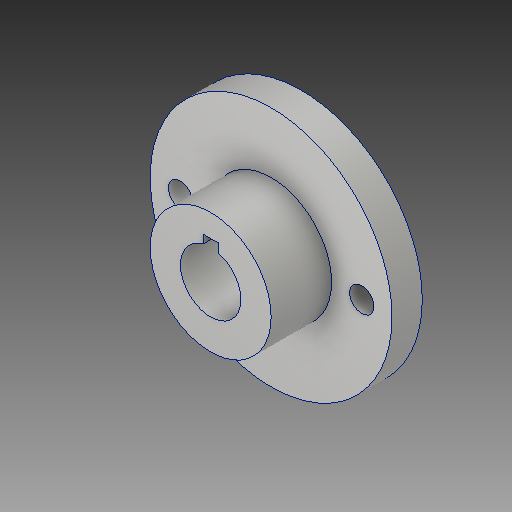
# Autodesk Inventor part: Hub Connected to Steel Tubing - 0.5in. Diameter
Saved by Autodesk Inventor 2019 (Build 230136000, 136)
## iProperties
Created: 2018-11-13
Part Number: Hub Connected to Steel Tubing - 0.5in. Diameter
Material: Aluminum 6061
Document SubType Name: Modeling
Designer: Alex Barnett
Density: 2.7 g/cm^3
Appearance: Aluminum - Flat
Mass: 44.6442 g
Surface Area: 67.6582 cm^2
Volume: 16.5349 cm^3
Author: Alex Barnett
Autodesk Inventor part; units mm, degrees
ref_plane "YZ Plane" through (0, 0, 0) normal (1, 0, 0) x (0, 1, 0)
ref_plane "XZ Plane" through (0, 0, 0) normal (0, 1, 0) x (-1, 0, 0)
ref_plane "XY Plane" through (0, 0, 0) normal (0, 0, 1) x (1, 0, 0)
sketch "Sketch1" plane through (0, 0, 0) normal (0, 0, 1) x (1, 0, 0)
  circle A0 centre (0, 0) radius 6.35
  circle A1 centre (0, 0) radius 25.4
  dimension "d0" = 12.7
  dimension "d1" = 50.8
  constraints: 2 centre point, 2 coincident
  measures "d0" diameter of A0
  measures "d1" diameter of A1
extrude "Extrusion1" add sketch "Sketch1" along normal blind 6.35
sketch "Sketch2" plane through (0, 0, 6.35) normal (0, 0, 1) x (1, 0, 0)
  circle A0 centre (0, 0) radius 6.35
  circle A1 centre (0, 0) radius 12.7
  dimension "d4" = 12.7
  dimension "d5" = 25.4
  constraints: 2 centre point, 2 coincident
  measures "d4" diameter of A0
  measures "d5" diameter of A1
extrude "Extrusion2" add sketch "Sketch2" along normal blind 12.7
sketch "Sketch3" plane through (0, 0, 19.05) normal (0, 0, 1) x (1, 0, 0)
  circle A0 centre (0, 0) radius 6.35 projected
  circle A1 centre (0, 0) radius 12.7 projected
  line L0 (1.5875, 4.7625) -> (-1.5875, 4.7625)
  line L1 (-1.5875, 4.7625) -> (-1.5875, 7.9375)
  line L2 (-1.5875, 7.9375) -> (1.5875, 7.9375)
  line L3 (1.5875, 7.9375) -> (1.5875, 4.7625)
  line L4 (1.5875, 4.7625) -> (-1.5875, 7.9375) construction
  line L5 (-1.5875, 4.7625) -> (1.5875, 7.9375) construction
  point P0 (0, 6.35)
  dimension "d8" = 3.175
  dimension "d9" = 3.175
  constraints: 12 end point, 2 midpoint, 2 parallel, 1 horizontal, 1 perpendicular, 1 vertical alignment, 1 other
  measures "d8" distance of L1.end L2.end
  measures "d9" distance of L0.end L1.end
extrude "Extrusion3" cut sketch "Sketch3" against normal blind 25.4 contours L3 L0 L1 A0 | A0 L1 L2 L3 picked at (0.1781, 5.2842)
sketch "Sketch4" plane through (0, 0, 6.35) normal (0, 0, 1) x (1, 0, 0)
  circle A0 centre (0, 0) radius 12.7 projected
  circle A1 centre (0, 0) radius 25.4 projected
  circle A2 centre (0, 0) radius 19.05 construction
  circle A3 centre (-19.05, 0) radius 2.413
  circle A4 centre (19.05, 0) radius 2.413
  dimension "d12" = 38.1
  dimension "d13" = 4.826
  dimension "d14" = 4.826
  constraints: 3 centre point, 2 point on circle, 1 coincident
  measures "d12" diameter of A2
  measures "d13" diameter of A3
  measures "d14" diameter of A4
hole "Hole1" at (-19.05, 0, 6.35) at (19.05, 0, 6.35) direction (0, 0, -1) diameter 5.08 end through all
body "Solid1"
